Autodesk Fusion 360 part; units mm, degrees
(part 3 of 3)
sketch "スケッチ5 (2)" plane through (0, 0, 0) normal (0, 0, 1) x (1, 0, 0) in component "新型ホイール v3"
  line L0 (0, -10) -> (0, -7)
  line L1 (0, -7) -> (-2.5, -7)
  line L2 (-2.5, -7) -> (2.5, -7)
  line L3 (2.5, -7) -> (2.5, -5)
  line L4 (2.5, -5) -> (-2.5, -5)
  line L5 (-2.5, -5) -> (-2.5, -7)
  line L6 (0, -10) -> (0.496, -10)
  dimension "d18" = 2.5
  dimension "d19" = 5
  dimension "d20" = 2
  constraint vertical L0
  constraint perpendicular L0 L1
  constraint horizontal L2
  constraint vertical L3
  constraint horizontal L4
  constraint vertical L5
  constraint perpendicular L0 L6
  measures "d18" distance of L0.end L1.end
  measures "d19" distance of L1.end L2.end
  measures "d20" distance of L1.end L4.end
revolve "回転4" add sketch "スケッチ5 (2)" angle 360 about axis through (0, -10, 0) along (1, 0, 0) separate body makes body 4 in component "新型ホイール v3"
move_body "移動6" bodies 4 to x (1, 0, 0) y (0, 1, 0) z (0, 0, 1) at (0, 10, 0) in component "新型ホイール v3"
sketch "スケッチ1 (3)" plane through (0, 0, 0) normal (1, 0, 0) x (0, 1, 0) in component "ワッシャー v2"
  circle A0 centre (0, 0) radius 1
  dimension "d1_1" = 2
  constraint coincident A0.centre origin
  measures "d1_1" diameter of A0
sketch "スケッチ2 (2)" plane through (0, 0, 0) normal (0, 1, 0) x (1, 0, 0) in component "ワッシャー v2"
  line L0 (0, -1) -> (-0.5, -1)
  line L1 (-0.5, -1) -> (-0.5, -4)
  line L2 (0, -1) -> (0.5, -1)
  line L3 (0.5, -1) -> (0.5, -4)
  line L4 (0.5, -4) -> (-0.5, -4)
  dimension "d2_2" = 3
  constraint horizontal L0
  constraint perpendicular L0 L1
  constraint parallel L0 L2
  constraint perpendicular L0 L3
  measures "d2_2" distance of L0.end L1.end
revolve "回転1'" add sketch "スケッチ2 (2)" angle 360 about axis through (1.75, 0, 0) along (1, 0, 0) separate body makes body 5 in component "ワッシャー v2"
extrude "押し出し1" cut 1 faces at (0.5, -2.4715, 1.6873) along direction (-1, 0, 0) blind 0.5 on bodies 5 bodies 5 in component "ワッシャー v2"
sketch "スケッチ1 (4)" plane through (0, 0, 0) normal (1, 0, 0) x (0, 1, 0) in component "ワッシャー v2 (1)"
  circle A0 centre (0, 0) radius 1
  dimension "d1_2" = 2
  constraint coincident A0.centre origin
  measures "d1_2" diameter of A0
sketch "スケッチ2 (3)" plane through (0, 0, 0) normal (0, 1, 0) x (1, 0, 0) in component "ワッシャー v2 (1)"
  line L0 (0, -1) -> (-0.5, -1)
  line L1 (-0.5, -1) -> (-0.5, -4)
  line L2 (0, -1) -> (0.5, -1)
  line L3 (0.5, -1) -> (0.5, -4)
  line L4 (0.5, -4) -> (-0.5, -4)
  dimension "d2_3" = 3
  constraint horizontal L0
  constraint perpendicular L0 L1
  constraint parallel L0 L2
  constraint perpendicular L0 L3
  measures "d2_3" distance of L0.end L1.end
revolve "回転1''" add sketch "スケッチ2 (3)" angle 360 about axis through (1.75, 0, 0) along (1, 0, 0) separate body makes body 6 in component "ワッシャー v2 (1)"
extrude "押し出し1'" cut 1 faces at (0.5, -2.4715, 1.6873) along direction (-1, 0, 0) blind 0.5 on bodies 6 bodies 6 in component "ワッシャー v2 (1)"
sketch "スケッチ6" plane through (0, 0, 0) normal (0, 0, 1) x (1, 0, 0) in component "新型ホイール v3"
component_pattern "component pattern"
component "新型ホイール v3" placed x (0, 0, 1) y (0, 1, 0) z (-1, 0, 0) at (22.5, 0, 0)
component "新型ホイール v3" placed x (0.5, 0, 0.866025) y (0, 1, 0) z (-0.866025, 0, 0.5) at (19.4856, 0, -11.25)
component "新型ホイール v3" placed x (0.866025, 0, 0.5) y (0, 1, 0) z (-0.5, 0, 0.866025) at (11.25, 0, -19.4856)
component "新型ホイール v3" placed x (1, 0, 0) y (0, 1, 0) z (0, 0, 1) at (0, 0, -22.5)
component "新型ホイール v3" placed x (0.866025, 0, -0.5) y (0, 1, 0) z (0.5, 0, 0.866025) at (-11.25, 0, -19.4856)
component "新型ホイール v3" placed x (0.5, 0, -0.866025) y (0, 1, 0) z (0.866025, 0, 0.5) at (-19.4856, 0, -11.25)
component "新型ホイール v3" placed x (0, 0, -1) y (0, 1, 0) z (1, 0, 0) at (-22.5, 0, 0)
component "新型ホイール v3" placed x (-0.5, 0, -0.866025) y (0, 1, 0) z (0.866025, 0, -0.5) at (-19.4856, 0, 11.25)
component "新型ホイール v3" placed x (-0.866025, 0, -0.5) y (0, 1, 0) z (0.5, 0, -0.866025) at (-11.25, 0, 19.4856)
component "新型ホイール v3" placed x (-1, 0, 0) y (0, 1, 0) z (0, 0, -1) at (0, 0, 22.5)
component "新型ホイール v3" placed x (-0.866025, 0, 0.5) y (0, 1, 0) z (-0.5, 0, -0.866025) at (11.25, 0, 19.4856)
component "新型ホイール v3" placed x (-0.5, 0, 0.866025) y (0, 1, 0) z (-0.866025, 0, -0.5) at (19.4856, 0, 11.25)
component "ワッシャー v2" placed x (1, 0, 0) y (0, 1, 0) z (0, 0, 1) at (3, 0, 0) in component "新型ホイール v3"
component "ワッシャー v2 (1)" placed x (1, 0, 0) y (0, 1, 0) z (0, 0, 1) at (-2.5, 0, 0) in component "新型ホイール v3"
